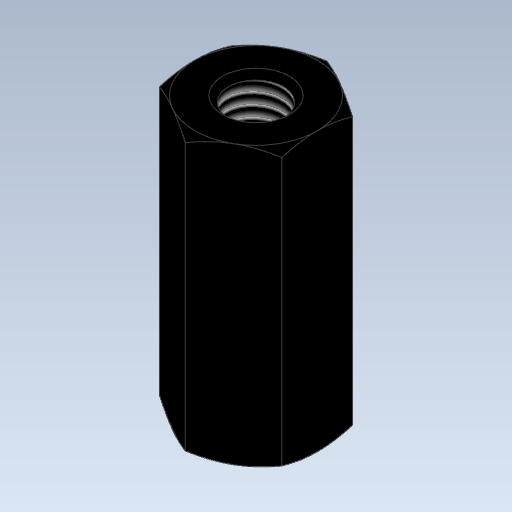
# Autodesk Inventor part: AS-312.5B
Saved by Autodesk Inventor 2020 (Build 240168000, 168)
## iProperties
Part Number: AS-312.5B
Material: アセタール樹脂、黒
Document SubType Name: Modeling
Designer: Masato Kubotera
Density: 2.7065 g/cm^3
Appearance: 黒
Catalog Web Link: https://www.hirosugi-net.co.jp/shop/g/g4377/
Description: ReadyMade
Mass: 0.723 g
Surface Area: 3.72905 cm^2
Volume: 0.267135 cm^3
Author: Masato Kubotera
Comments: Width across flats : 5.5
Autodesk Inventor part; units mm, degrees
ref_plane "YZ Plane" through (0, 0, 0) normal (1, 0, 0) x (0, 1, 0)
ref_plane "XZ Plane" through (0, 0, 0) normal (0, 1, 0) x (-1, 0, 0)
ref_plane "XY Plane" through (0, 0, 0) normal (0, 0, 1) x (1, 0, 0)
sketch "スケッチ1" plane through (0, 0, 0) normal (1, 0, 0) x (0, 1, 0)
  line L0 (-6.25, 0) -> (6.25, 0)
  line L1 (0, 0) -> (0, 3.1754) construction
  line L2 (-6.0044, 3.1754) -> (-6.25, 2.75)
  line L3 (-6.25, 2.75) -> (-6.25, 0)
  line L4 (-6.0044, 3.1754) -> (6.0044, 3.1754)
  line L5 (6.0044, 3.1754) -> (6.25, 2.75)
  line L6 (6.25, 2.75) -> (6.25, 0)
  dimension "d1" = 2.75
  dimension "d2" = 3.1754
  dimension "d3" = 30
  dimension "d4" = 12.5
  constraints: 14 end point, 3 perpendicular, 2 midpoint, 1 coincident, 1 horizontal, 1 symmetric about line
  measures "d1" distance of L0.start L2.end
  measures "d2" vertical distance of L0.start L2.start
  measures "d3" angle of L3 L2
  measures "d4" distance of L0.start L0.end
revolve "回転1" add sketch "スケッチ1" angle 360 about axis through (0, -6.25, 0) along (0, 1, 0)
sketch "スケッチ2" plane through (0, 6.25, 0) normal (0, 1, 0) x (1, 0, 0)
  line L0 (0, -3.1754) -> (-2.75, -1.5877)
  line L1 (-2.75, -1.5877) -> (-2.75, 1.5877)
  line L2 (-2.75, 1.5877) -> (0, 3.1754)
  line L3 (0, 3.1754) -> (2.75, 1.5877)
  line L4 (2.75, 1.5877) -> (2.75, -1.5877)
  line L5 (2.75, -1.5877) -> (0, -3.1754)
  circle A0 centre (0, 0) radius 3.1754 projected
  point P0 (0, 0)
  point P1 (0, 0)
  point P2 (0, 0)
  point P3 (0, 0)
  point P4 (0, 3.1754)
  point P5 (0, 3.1754)
  point P6 (2.75, -1.5877)
  point P7 (2.75, -1.5877)
  constraints: 12 end point, 2 coincident, 1 vertical, 15 other
extrude "押し出し1" cut sketch "スケッチ2" against normal through all contours A0 L0 | L5 A0 | A0 L1 | L4 A0 | A0 L2 | L3 A0
hole "穴1" at (0, 6.25, 0) direction (0, -1, 0) diameter 2.459 end through all countersink diameter 3 countersink angle 90 thread size "M3x0.5" class "6H" standard "ISO Metric profile"
mirror "ミラー1" about plane through (0, 0, 0) normal (0, 1, 0) of "穴1"
equation "\"d2\" = 1.1547 * d1"
